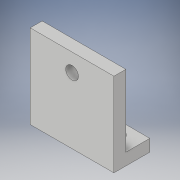
# Autodesk Inventor part: AngleBracketForEndOfArm
Saved by Autodesk Inventor 2017 SP1 (Build 210196100, 196)
## iProperties
Created: 2016-08-17
Part Number: AngleBracketForEndOfArm
Material: Generic
Document SubType Name: Modeling
Designer: steele
Density: 1 g/cm^3
Appearance: Default
Author: steele
Autodesk Inventor part; units mm, degrees
ref_plane "YZ Plane" through (0, 0, 0) normal (1, 0, 0) x (0, 1, 0)
ref_plane "XZ Plane" through (0, 0, 0) normal (0, 1, 0) x (-1, 0, 0)
ref_plane "XY Plane" through (0, 0, 0) normal (0, 0, 1) x (1, 0, 0)
sketch "Sketch1" plane through (0, 0, 0) normal (1, 0, 0) x (0, 1, 0)
  line L0 (0, 0) -> (44.45, 0)
  line L1 (44.45, 0) -> (44.45, -6.35)
  line L2 (44.45, -6.35) -> (6.35, -6.35)
  line L3 (6.35, -6.35) -> (6.35, -19.05)
  line L4 (6.35, -19.05) -> (0, -19.05)
  line L5 (0, -19.05) -> (0, 0)
  dimension "d0" = 6.35
  dimension "d1" = 44.45
  dimension "d21" = 19.05
  constraints: 12 end point, 6 perpendicular, 1 horizontal
  measures "d0" distance of L0.end L1.end
  measures "d1" distance of L0.start L0.end
  measures "d21" distance of L4.end L0.start
extrude "Extrusion1" add sketch "Sketch1" along normal blind 44.45
sketch "Sketch2" plane through (0, 0, 0) normal (0, 0, 1) x (1, 0, 0)
  line L0 (0, 44.45) -> (44.45, 44.45) construction
  line L1 (22.225, 44.45) -> (22.225, 0) construction
  line L2 (0, 0) -> (44.45, 0) construction
  point P0 (22.225, 34.925)
  dimension "d4" = 9.525
  constraints: 2 end point, 2 midpoint, 1 point on line
  measures "d4" distance from line of point (22.225, 34.925) L0
hole "Hole1" at (22.225, 34.925, 0) direction (0, 0, -1) diameter 6.7564 end through all clearance for "Flat Head Machine Screw (82)" size "1/4" standard "Ansi Unified Screw Threads"
sketch "Sketch4" plane through (0, 6.35, -6.35) normal (0, 1, 0) x (1, 0, 0)
  line L0 (0, 6.35) -> (44.45, 6.35) construction
  line L1 (44.45, -6.35) -> (44.45, 12.7) construction
  line L2 (0, 12.7) -> (44.45, 12.7) projected
  line L3 (0, 0) -> (0, 12.7) projected
  point P0 (0, -6.35)
  point P1 (22.225, 6.35)
  point P2 (9.525, 6.35)
  point P3 (34.925, 6.35)
  dimension "d22" = 6.35
  dimension "d23" = 9.525
  dimension "d24" = 9.525
  constraints: 3 point on line, 2 end point, 1 horizontal, 1 midpoint
  measures "d22" distance between parallel lines of L2 L0
  measures "d23" distance from line of L3 point (9.525, 6.35)
  measures "d24" distance from line of point (34.925, 6.35) L1
hole "Hole3" at (22.225, 6.35, -12.7) at (9.525, 6.35, -12.7) at (34.925, 6.35, -12.7) direction (0, -1, 0) diameter 5.1054 end through all clearance for "Flat Head Machine Screw (82)" size "#10" standard "Ansi Unified Screw Threads"
body "Solid1"
